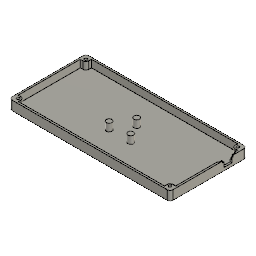
Keyboard Housing (Autodesk Fusion 360 design; units mm, degrees)
Autodesk Fusion 360 part; units mm, degrees
sketch "Sketch1" plane through (0, 0, 0) normal (0, 0, 1) x (1, 0, 0)
  line L0 (8.2886, 10.0322) -> (8.2886, 86.7075)
  line L1 (178.4519, 7.0322) -> (11.2886, 7.0322)
  line L2 (181.4519, 86.7075) -> (181.4519, 10.0322)
  line L3 (11.2886, 89.7075) -> (178.4519, 89.7075)
  line L4 (8.2886, 89.7075) -> (181.4519, 89.7075)
  line L5 (181.4519, 89.7075) -> (181.4519, 7.0322)
  line L6 (181.4519, 7.0322) -> (8.2886, 7.0322)
  line L7 (8.2886, 7.0322) -> (8.2886, 89.7075)
  constraint horizontal L4
  constraint vertical L5
  constraint horizontal L6
  constraint vertical L7
extrude "Extrude1" add sketch "Sketch1" along normal blind 2
sketch "Sketch2" plane through (0, 0, 2) normal (0, 0, 1) x (-1, 0, 0)
  line L0 (-8.2886, -7.0322) -> (-181.4519, -7.0322)
  line L1 (-181.4519, -7.0322) -> (-181.4519, -89.7075)
  line L2 (-181.4519, -89.7075) -> (-8.2886, -89.7075)
  line L3 (-8.2886, -89.7075) -> (-8.2886, -7.0322)
  line L4 (-10.2886, -87.7075) -> (-179.4519, -87.7075)
  line L5 (-179.4519, -87.7075) -> (-179.4519, -9.0322)
  line L6 (-179.4519, -9.0322) -> (-10.2886, -9.0322)
  line L7 (-10.2886, -9.0322) -> (-10.2886, -87.7075)
  line L8 (-8.2886, -15.0322) -> (-13.2886, -15.0322)
  arc A0 (-16.2886, -12.0322) -> (-13.2886, -15.0322) centre (-13.2886, -12.0322) ccw
  line L9 (-16.2886, -12.0322) -> (-16.2886, -7.0322)
  circle A1 centre (-13.2886, -12.0322) radius 1.5
  line L10 (-16.2886, -89.7075) -> (-16.2886, -84.7075)
  arc A2 (-13.2886, -81.7075) -> (-16.2886, -84.7075) centre (-13.2886, -84.7075) ccw
  line L11 (-13.2886, -81.7075) -> (-8.2886, -81.7075)
  circle A3 centre (-13.2886, -84.7075) radius 1.5
  line L12 (-181.4519, -81.7075) -> (-176.4519, -81.7075)
  arc A4 (-173.4519, -84.7075) -> (-176.4519, -81.7075) centre (-176.4519, -84.7075) ccw
  line L13 (-173.4519, -84.7075) -> (-173.4519, -89.7075)
  circle A5 centre (-176.4519, -84.7075) radius 1.5
  line L14 (-181.4519, -15.0322) -> (-176.4519, -15.0322)
  arc A6 (-176.4519, -15.0322) -> (-173.4519, -12.0322) centre (-176.4519, -12.0322) ccw
  line L15 (-173.4519, -12.0322) -> (-173.4519, -7.0322)
  circle A7 centre (-176.4519, -12.0322) radius 1.5
  circle A8 centre (-83.2886, -39.7075) radius 3
  circle A9 centre (-106.4519, -39.7075) radius 3
  line L16 (-94.8702, -89.7075) -> (-94.8702, -57.7075) construction
  circle A10 centre (-94.8702, -57.7075) radius 3
  dimension "d128" = 2
  dimension "d129" = 2
  dimension "d130" = 2
  dimension "d131" = 2
  dimension "d132" = 5
  dimension "d133" = 5
  dimension "d134" = 3
  dimension "d135" = 3
  dimension "d136" = 5
  dimension "d137" = 3
  dimension "d138" = 5
  dimension "d139" = 3
  dimension "d140" = 5
  dimension "d141" = 5
  dimension "d142" = 3
  dimension "d143" = 3
  dimension "d144" = 5
  dimension "d145" = 5
  dimension "d146" = 3
  dimension "d147" = 3
  dimension "d150" = 6
  dimension "d151" = 6
  dimension "d152" = 50
  dimension "d153" = 75
  dimension "d154" = 50
  dimension "d155" = 75
  dimension "d156" = 32
  dimension "d157" = 6
  constraint horizontal L4
  constraint vertical L5
  constraint horizontal L6
  constraint vertical L7
  constraint coincident L3 L8.start
  constraint perpendicular L3 L8
  constraint tangent L8 A0
  constraint coincident L0 L9.end
  constraint perpendicular L0 L9
  constraint tangent A0 L9
  constraint concentric A0 A1
  constraint coincident L2 L10.start
  constraint perpendicular L2 L10
  constraint tangent L10 A2
  constraint coincident L3 L11.end
  constraint tangent A2 L11
  constraint perpendicular L3 L11
  constraint concentric A2 A3
  constraint coincident L1 L12.start
  constraint perpendicular L1 L12
  constraint tangent L12 A4
  constraint coincident L2 L13.end
  constraint perpendicular L2 L13
  constraint tangent A4 L13
  constraint concentric A4 A5
  constraint coincident L1 L14.start
  constraint perpendicular L1 L14
  constraint tangent L14 A6
  constraint coincident L0 L15.end
  constraint tangent A6 L15
  constraint perpendicular L0 L15
  constraint concentric A6 A7
  constraint midpoint L2 L16.start
  constraint perpendicular L2 L16
  constraint coincident L16.end A10.centre
  measures "d128" distance of L2 L4
  measures "d129" distance of L3 L7
  measures "d130" distance of L0 L6
  measures "d131" distance of L1 L5
  measures "d132" distance of L8.start L8.end
  measures "d133" distance of A0.start L9.end
  measures "d134" radius of A0
  measures "d135" diameter of A1
  measures "d136" distance of L10.start L10.end
  measures "d137" radius of A2
  measures "d138" distance of A2.start L11.end
  measures "d139" diameter of A3
  measures "d140" distance of L12.start L12.end
  measures "d141" distance of A4.start L13.end
  measures "d142" radius of A4
  measures "d143" diameter of A5
  measures "d144" distance of L14.start L14.end
  measures "d145" distance of A6.end L15.end
  measures "d146" radius of A6
  measures "d147" diameter of A7
  measures "d150" diameter of A8
  measures "d151" diameter of A9
  measures "d152" distance of L2 A8.centre
  measures "d153" distance of L3 A8.centre
  measures "d154" distance of L2 A9.centre
  measures "d155" distance of L1 A9.centre
  measures "d156" distance of L16.start L16.end
  measures "d157" diameter of A10
extrude "Extrude2" add sketch "Sketch2" along normal blind 8 contours L0 L3 L6 L7 L8 L9 | L0 L6 L9 L15 | L3 L7 L8 L11 | L0 L1 L5 L6 L14 L15 | L6 L7 L8 A0 L9 | L2 L3 L4 L7 L10 L11 | L5 L6 L14 A6 L15 | L4 L7 L10 A2 L11 | L1 L5 L12 L14 | L2 L4 L10 L13 | L1 L2 L4 L5 L12 L13 | L4 L5 L12 A4 L13 | A8 | A9 | A10
sketch "Sketch3" plane through (0, 0, 10) normal (0, 0, 1) x (-1, 0, 0)
  circle A0 centre (-13.2886, -12.0322) radius 1.5
  line L0 (-176.4519, -81.7075) -> (-179.4519, -81.7075)
  line L1 (-179.4519, -81.7075) -> (-179.4519, -15.0322)
  line L2 (-179.4519, -15.0322) -> (-176.4519, -15.0322)
  arc A1 (-176.4519, -15.0322) -> (-173.4519, -12.0322) centre (-176.4519, -12.0322) ccw
  line L3 (-173.4519, -12.0322) -> (-173.4519, -9.0322)
  line L4 (-173.4519, -9.0322) -> (-16.2886, -9.0322)
  line L5 (-16.2886, -9.0322) -> (-16.2886, -12.0322)
  arc A2 (-16.2886, -12.0322) -> (-13.2886, -15.0322) centre (-13.2886, -12.0322) ccw
  line L6 (-13.2886, -15.0322) -> (-10.2886, -15.0322)
  line L7 (-10.2886, -15.0322) -> (-10.2886, -81.7075)
  line L8 (-10.2886, -81.7075) -> (-13.2886, -81.7075)
  arc A3 (-13.2886, -81.7075) -> (-16.2886, -84.7075) centre (-13.2886, -84.7075) ccw
  line L9 (-16.2886, -84.7075) -> (-16.2886, -87.7075)
  line L10 (-16.2886, -87.7075) -> (-173.4519, -87.7075)
  line L11 (-173.4519, -87.7075) -> (-173.4519, -84.7075)
  arc A4 (-173.4519, -84.7075) -> (-176.4519, -81.7075) centre (-176.4519, -84.7075) ccw
  circle A5 centre (-176.4519, -84.7075) radius 1.5
  circle A6 centre (-176.4519, -12.0322) radius 1.5
  circle A7 centre (-13.2886, -84.7075) radius 1.5
  line L12 (-8.2886, -89.7075) -> (-8.2886, -7.0322)
  line L13 (-8.2886, -7.0322) -> (-181.4519, -7.0322)
  line L14 (-181.4519, -7.0322) -> (-181.4519, -89.7075)
  line L15 (-181.4519, -89.7075) -> (-8.2886, -89.7075)
  line L16 (-179.4519, -74.9075) -> (-181.4519, -74.9075)
  line L17 (-181.4519, -74.9075) -> (-181.4519, -63.5075)
  line L18 (-181.4519, -63.5075) -> (-179.4519, -63.5075)
  line L19 (-179.4519, -63.5075) -> (-179.4519, -74.9075)
  dimension "d158" = 11.4
  dimension "d159" = 14.8
  constraint horizontal L16
  constraint vertical L17
  constraint horizontal L18
  constraint vertical L19
  constraint coincident L14 L17.end
  constraint coincident L1 L16.start
  measures "d158" distance of L16 L18
  measures "d159" distance of L15 L16
extrude "Extrude3" cut sketch "Sketch3" against normal blind 1.7 contours L1 L14 L16 L17 L18 L19
sketch "Sketch4" plane through (0, 0, 8.3) normal (0, 0, 1) x (-1, 0, 0)
  line L0 (-179.4519, -63.5075) -> (-181.4519, -63.5075)
  line L1 (-181.4519, -63.5075) -> (-181.4519, -74.9075)
  line L2 (-181.4519, -74.9075) -> (-179.4519, -74.9075)
  line L3 (-179.4519, -74.9075) -> (-179.4519, -63.5075)
  line L4 (-179.4519, -73.4575) -> (-181.4519, -73.4575)
  line L5 (-181.4519, -73.4575) -> (-181.4519, -64.9575)
  line L6 (-181.4519, -64.9575) -> (-179.4519, -64.9575)
  line L7 (-179.4519, -64.9575) -> (-179.4519, -73.4575)
  dimension "d162" = 8.5
  constraint horizontal L4
  constraint vertical L5
  constraint horizontal L6
  constraint vertical L7
  constraint coincident L1 L5.end
  constraint coincident L3 L4.start
  constraint midpoint L3 L7
  measures "d162" distance of L4.end L5.end
extrude "Extrude4" cut sketch "Sketch4" against normal blind 5 contours L1 L3 L4 L5 L6 L7
fillet "Fillet1" radius 3 4 edges at (8.2886, 7.0322, 5) (8.2886, 89.7075, 5) (181.4519, 7.0322, 5) (181.4519, 89.7075, 5)
sketch "Sketch5" plane through (0, 0, 10) normal (0, 0, 1) x (-1, 0, 0)
  circle A0 centre (-176.4519, -12.0322) radius 1.5
  arc A1 (-181.4519, -86.7075) -> (-178.4519, -89.7075) centre (-178.4519, -86.7075) ccw
  line L0 (-178.4519, -89.7075) -> (-11.2886, -89.7075)
  arc A2 (-11.2886, -89.7075) -> (-8.2886, -86.7075) centre (-11.2886, -86.7075) ccw
  line L1 (-8.2886, -86.7075) -> (-8.2886, -10.0322)
  arc A3 (-8.2886, -10.0322) -> (-11.2886, -7.0322) centre (-11.2886, -10.0322) ccw
  line L2 (-11.2886, -7.0322) -> (-178.4519, -7.0322)
  arc A4 (-178.4519, -7.0322) -> (-181.4519, -10.0322) centre (-178.4519, -10.0322) ccw
  line L3 (-181.4519, -10.0322) -> (-181.4519, -63.5075)
  line L4 (-181.4519, -63.5075) -> (-179.4519, -63.5075)
  line L5 (-179.4519, -63.5075) -> (-179.4519, -15.0322)
  line L6 (-179.4519, -15.0322) -> (-176.4519, -15.0322)
  arc A5 (-176.4519, -15.0322) -> (-173.4519, -12.0322) centre (-176.4519, -12.0322) ccw
  line L7 (-173.4519, -12.0322) -> (-173.4519, -9.0322)
  line L8 (-173.4519, -9.0322) -> (-16.2886, -9.0322)
  line L9 (-16.2886, -9.0322) -> (-16.2886, -12.0322)
  arc A6 (-16.2886, -12.0322) -> (-13.2886, -15.0322) centre (-13.2886, -12.0322) ccw
  line L10 (-13.2886, -15.0322) -> (-10.2886, -15.0322)
  line L11 (-10.2886, -15.0322) -> (-10.2886, -81.7075)
  line L12 (-10.2886, -81.7075) -> (-13.2886, -81.7075)
  arc A7 (-13.2886, -81.7075) -> (-16.2886, -84.7075) centre (-13.2886, -84.7075) ccw
  line L13 (-16.2886, -84.7075) -> (-16.2886, -87.7075)
  line L14 (-16.2886, -87.7075) -> (-173.4519, -87.7075)
  line L15 (-173.4519, -87.7075) -> (-173.4519, -84.7075)
  arc A8 (-173.4519, -84.7075) -> (-176.4519, -81.7075) centre (-176.4519, -84.7075) ccw
  line L16 (-176.4519, -81.7075) -> (-179.4519, -81.7075)
  line L17 (-179.4519, -81.7075) -> (-179.4519, -74.9075)
  line L18 (-179.4519, -74.9075) -> (-181.4519, -74.9075)
  line L19 (-181.4519, -74.9075) -> (-181.4519, -86.7075)
  circle A9 centre (-13.2886, -84.7075) radius 1.5
  circle A10 centre (-13.2886, -12.0322) radius 1.5
  circle A11 centre (-176.4519, -84.7075) radius 1.5
  line L20 (-179.4519, -78.2075) -> (-180.4519, -78.2075)
  line L21 (-180.4519, -78.2075) -> (-180.4519, -60.2075)
  line L22 (-180.4519, -60.2075) -> (-179.4519, -60.2075)
  line L23 (-179.4519, -60.2075) -> (-179.4519, -78.2075)
  line L24 (-179.4519, -64.9575) -> (-179.4519, -73.4575)
  dimension "d166" = 18
  dimension "d167" = 1
  constraint horizontal L20
  constraint vertical L21
  constraint horizontal L22
  constraint vertical L23
  constraint coincident L17 L20.start
  constraint midpoint L23 L24
  measures "d166" distance of L20.start L22.end
  measures "d167" distance of L20.start L20.end
extrude "Extrude5" cut sketch "Sketch5" against normal blind 4 contours L4 L18 L21 L23 L24 | L17 L18 L20 L21 L23 | L4 L5 L21 L22 L23
